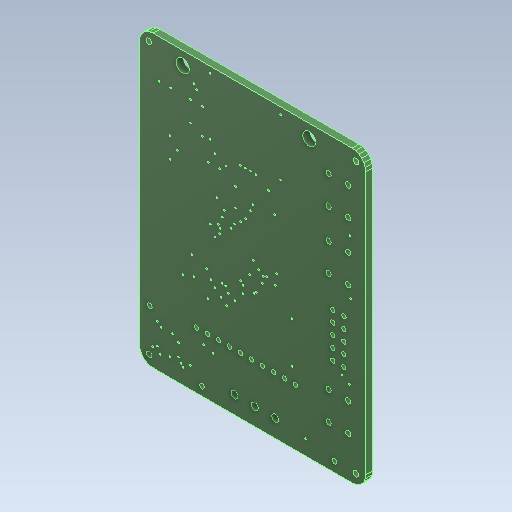
# Autodesk Inventor part: BLE Board.brd_Outline
Saved by Autodesk Inventor 2021 (Build 250183000, 183)
## iProperties
Created: 2020-11-03
Part Number: BLE Board.brd_Outline
Material: Generic
Document SubType Name: Modeling
Designer: faiya
Density: 1 g/cm^3
Appearance: Board Outline
Author: faiya
Autodesk Inventor part; units mm, degrees
ref_plane "YZ Plane" through (0, 0, 0) normal (1, 0, 0) x (0, 1, 0)
ref_plane "XZ Plane" through (0, 0, 0) normal (0, 1, 0) x (-1, 0, 0)
ref_plane "XY Plane" through (0, 0, 0) normal (0, 0, 1) x (1, 0, 0)
sketch "Sketch1" plane through (0, 0, 0) normal (0, 0, 1) x (1, 0, 0)
  line L0 (-6.604, 63.805) -> (-6.604, 3.175)
  line L1 (-6.604, 3.175) -> (-6.4958, 2.3533)
  line L2 (-6.4958, 2.3533) -> (-6.1786, 1.5875)
  line L3 (-6.1786, 1.5875) -> (-5.6741, 0.9299)
  line L4 (-5.6741, 0.9299) -> (-5.0165, 0.4254)
  line L5 (-5.0165, 0.4254) -> (-4.2508, 0.1082)
  line L6 (-4.2508, 0.1082) -> (-3.429, 0)
  line L7 (-3.429, 0) -> (42.525, 0)
  line L8 (42.525, 0) -> (43.3468, 0.1082)
  line L9 (43.3468, 0.1082) -> (44.1125, 0.4254)
  line L10 (44.1125, 0.4254) -> (44.7701, 0.9299)
  line L11 (44.7701, 0.9299) -> (45.2746, 1.5875)
  line L12 (45.2746, 1.5875) -> (45.5918, 2.3533)
  line L13 (45.5918, 2.3533) -> (45.7, 3.175)
  line L14 (45.7, 3.175) -> (45.7, 63.805)
  line L15 (45.7, 63.805) -> (45.5918, 64.6268)
  line L16 (45.5918, 64.6268) -> (45.2746, 65.3925)
  line L17 (45.2746, 65.3925) -> (44.7701, 66.0501)
  line L18 (44.7701, 66.0501) -> (44.1125, 66.5546)
  line L19 (44.1125, 66.5546) -> (43.3468, 66.8718)
  line L20 (43.3468, 66.8718) -> (42.525, 66.98)
  line L21 (42.525, 66.98) -> (-3.429, 66.98)
  line L22 (-3.429, 66.98) -> (-4.2508, 66.8718)
  line L23 (-4.2508, 66.8718) -> (-5.0165, 66.5546)
  line L24 (-5.0165, 66.5546) -> (-5.6741, 66.0501)
  line L25 (-5.6741, 66.0501) -> (-6.1786, 65.3925)
  line L26 (-6.1786, 65.3925) -> (-6.4958, 64.6268)
  line L27 (-6.4958, 64.6268) -> (-6.604, 63.805)
  circle A0 centre (7.87, 2.03) radius 0.55
  circle A1 centre (38.48, 2.29) radius 0.55
  circle A2 centre (6.6, 13.08) radius 0.5
  circle A3 centre (9.14, 13.08) radius 0.5
  circle A4 centre (11.68, 13.08) radius 0.5
  circle A5 centre (14.22, 13.08) radius 0.5
  circle A6 centre (16.76, 13.08) radius 0.5
  circle A7 centre (19.3, 13.08) radius 0.5
  circle A8 centre (21.84, 13.08) radius 0.5
  circle A9 centre (24.38, 13.08) radius 0.5
  circle A10 centre (26.92, 13.08) radius 0.5
  circle A11 centre (29.46, 13.08) radius 0.5
  circle A12 centre (-4.19, 12.07) radius 0.55
  circle A13 centre (38.1, 27.3) radius 0.5
  circle A14 centre (38.1, 29.85) radius 0.5
  circle A15 centre (38.1, 32.38) radius 0.5
  circle A16 centre (40.64, 32.38) radius 0.5
  circle A17 centre (38.1, 24.77) radius 0.5
  circle A18 centre (40.64, 22.23) radius 0.5
  circle A19 centre (40.64, 29.85) radius 0.5
  circle A20 centre (40.64, 27.3) radius 0.5
  circle A21 centre (40.64, 24.77) radius 0.5
  circle A22 centre (38.1, 22.23) radius 0.5
  circle A23 centre (15.37, 4.06) radius 0.8
  circle A24 centre (20.07, 4.06) radius 0.8
  circle A25 centre (24.77, 4.06) radius 0.8
  circle A26 centre (37.11, 15.95) radius 0.6
  circle A27 centre (37.11, 9.45) radius 0.6
  circle A28 centre (41.63, 15.95) radius 0.6
  circle A29 centre (41.63, 9.45) radius 0.6
  circle A30 centre (41.63, 52.63) radius 0.6
  circle A31 centre (41.63, 59.13) radius 0.6
  circle A32 centre (37.11, 52.63) radius 0.6
  circle A33 centre (37.11, 59.13) radius 0.6
  circle A34 centre (41.63, 39.17) radius 0.6
  circle A35 centre (41.63, 45.67) radius 0.6
  circle A36 centre (37.11, 39.17) radius 0.6
  circle A37 centre (37.11, 45.67) radius 0.6
  circle A38 centre (-4.4196, 64.8462) radius 0.635
  circle A39 centre (43.434, 64.77) radius 0.635
  circle A40 centre (-4.318, 2.286) radius 0.635
  circle A41 centre (43.434, 2.286) radius 0.635
  circle A42 centre (3.429, 63.881) radius 1.5
  circle A43 centre (32.639, 63.881) radius 1.5
  circle A44 centre (9.2456, 20.2184) radius 0.1905
  circle A45 centre (13.335, 24.765) radius 0.1905
  circle A46 centre (13.462, 48.8652) radius 0.1905
  circle A47 centre (9.779, 35.433) radius 0.1905
  circle A48 centre (11.938, 34.544) radius 0.1905
  circle A49 centre (20.9619, 31.8701) radius 0.1905
  circle A50 centre (19.7092, 33.147) radius 0.1905
  circle A51 centre (18.8664, 29.7746) radius 0.1905
  circle A52 centre (2.4638, 8.0772) radius 0.1905
  circle A53 centre (2.4384, 5.1308) radius 0.1905
  circle A54 centre (40.259, 20.447) radius 0.1905
  circle A55 centre (5.207, 4.826) radius 0.1905
  circle A56 centre (31.75, 3.429) radius 0.1905
  circle A57 centre (0.4826, 48.4124) radius 0.1905
  circle A58 centre (0.508, 43.7631) radius 0.1905
  circle A59 centre (10.922, 33.401) radius 0.1905
  circle A60 centre (5.969, 61.595) radius 0.1905
  circle A61 centre (9.906, 24.363) radius 0.1905
  circle A62 centre (12.319, 21.971) radius 0.1905
  circle A63 centre (13.97, 23.622) radius 0.1905
  circle A64 centre (20.4357, 27.0397) radius 0.1905
  circle A65 centre (9.779, 52.324) radius 0.1905
  circle A66 centre (26.035, 65.405) radius 0.1905
  circle A67 centre (26.035, 52.324) radius 0.1905
  circle A68 centre (9.779, 65.532) radius 0.1905
  circle A69 centre (10.922, 50.038) radius 0.1905
  circle A70 centre (23.241, 48.8398) radius 0.1905
  circle A71 centre (13.0048, 39.8018) radius 0.1905
  circle A72 centre (15.378, 38.216) radius 0.1905
  circle A73 centre (14.6033, 36.9587) radius 0.1905
  circle A74 centre (24.638, 44.704) radius 0.1905
  circle A75 centre (28.702, 16.383) radius 0.1905
  circle A76 centre (-1.5748, 9.0932) radius 0.1905
  circle A77 centre (1.016, 9.0678) radius 0.1905
  circle A78 centre (8.2804, 10.5156) radius 0.1905
  circle A79 centre (10.4394, 9.8806) radius 0.1905
  circle A80 centre (42.2275, 36.6395) radius 0.1905
  circle A81 centre (42.037, 49.149) radius 0.1905
  circle A82 centre (11.3538, 41.4528) radius 0.1905
  circle A83 centre (28.6766, 25.908) radius 0.1905
  circle A84 centre (-2.4638, 9.8552) radius 0.1905
  circle A85 centre (-2.4638, 4.9022) radius 0.1905
  circle A86 centre (-1.778, 3.4798) radius 0.1905
  circle A87 centre (3.556, 3.556) radius 0.1905
  circle A88 centre (17.272, 25.273) radius 0.1905
  circle A89 centre (15.621, 45.847) radius 0.1905
  circle A90 centre (15.621, 41.529) radius 0.1905
  circle A91 centre (12.573, 38.227) radius 0.1905
  circle A92 centre (-3.556, 4.204) radius 0.1905
  circle A93 centre (0.508, 4.191) radius 0.1905
  circle A94 centre (3.048, 4.191) radius 0.1905
  circle A95 centre (6.604, 60.706) radius 0.1905
  circle A96 centre (2.159, 46.355) radius 0.1905
  circle A97 centre (19.939, 26.543) radius 0.1905
  circle A98 centre (41.91, 19.431) radius 0.1905
  circle A99 centre (3.4798, 22.1488) radius 0.1905
  circle A100 centre (5.588, 27.178) radius 0.1905
  circle A101 centre (21.844, 29.591) radius 0.1905
  circle A102 centre (5.207, 53.34) radius 0.1905
  circle A103 centre (5.207, 58.039) radius 0.1905
  circle A104 centre (0.635, 58.039) radius 0.1905
  circle A105 centre (-2.032, 58.039) radius 0.1905
  circle A106 centre (11.938, 47.5742) radius 0.1905
  circle A107 centre (9.3472, 47.5488) radius 0.1905
  circle A108 centre (8.001, 58.039) radius 0.1905
  circle A109 centre (8.001, 52.07) radius 0.1905
  circle A110 centre (22.098, 31.115) radius 0.1905
  circle A111 centre (25.146, 33.147) radius 0.1905
  circle A112 centre (24.8154, 30.6574) radius 0.1905
  circle A113 centre (6.0198, 23.0124) radius 0.1905
  circle A114 centre (8.9662, 26.0096) radius 0.1905
  circle A115 centre (22.8117, 31.369) radius 0.1905
  circle A116 centre (17.907, 50.673) radius 0.1905
  circle A117 centre (17.907, 40.513) radius 0.1905
  circle A118 centre (17.399, 26.924) radius 0.1905
  circle A119 centre (16.764, 50.673) radius 0.1905
  circle A120 centre (16.764, 39.37) radius 0.1905
  circle A121 centre (16.764, 27.559) radius 0.1905
  circle A122 centre (11.684, 36.322) radius 0.1905
  circle A123 centre (19.6386, 44.196) radius 0.1905
  circle A124 centre (20.32, 50.5924) radius 0.1905
  circle A125 centre (12.065, 35.687) radius 0.1905
  circle A126 centre (19.05, 42.672) radius 0.1905
  circle A127 centre (19.05, 50.673) radius 0.1905
  circle A128 centre (10.8712, 23.241) radius 0.1905
  circle A129 centre (12.5407, 24.9105) radius 0.1905
  circle A130 centre (13.589, 20.955) radius 0.1905
  circle A131 centre (15.494, 22.86) radius 0.1905
  constraints: 132 centre point, 56 end point
extrude "BLE Board.brd_Outline" add sketch "Sketch1" along normal blind 1.6
body "Solid1"
